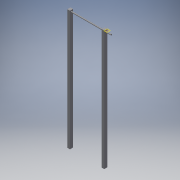
# Autodesk Inventor part: antebrazo
Saved by Autodesk Inventor 2016 (Build 200138000, 138)
## iProperties
Created: 2016-07-27
Part Number: antebrazo
Material: Generic
Document SubType Name: Modeling
Designer: Admin
Density: 1 g/cm^3
Appearance: Default
Author: Admin
Autodesk Inventor part; units mm, degrees
ref_plane "YZ Plane" through (0, 0, 0) normal (1, 0, 0) x (0, 1, 0)
ref_plane "XZ Plane" through (0, 0, 0) normal (0, 1, 0) x (-1, 0, 0)
ref_plane "XY Plane" through (0, 0, 0) normal (0, 0, 1) x (1, 0, 0)
ref_plane "Work Plane1" through (816103.6043, 395739.5889, 5886.7052) normal (0, 0, 1) x (1, 0, 0)
sketch "Sketch1" plane through (816103.6043, 395739.5889, 5886.7052) normal (0, 0, 1) x (1, 0, 0)
  line L0 (-6, 7) -> (-16, 7)
  line L1 (-16, 7) -> (-16, -5)
  line L2 (-16, -5) -> (-6, -5)
  line L3 (-6, -5) -> (-6, 7)
  line L4 (-144.5049, 7) -> (-134.5049, 7)
  line L5 (-134.5049, 7) -> (-134.5049, -5)
  line L6 (-134.5049, -5) -> (-144.5049, -5)
  line L7 (-144.5049, -5) -> (-144.5049, 7)
  point P0 (-816103.6043, -395739.5889)
  dimension "d0" = 10
  dimension "d1" = 12
  dimension "d2" = 10
  dimension "d3" = 12
  constraints: 16 end point, 4 parallel, 2 horizontal, 2 perpendicular, 1 point on line
  measures "d0" distance of L2.end L1.end
  measures "d1" distance of L1.end L0.end
  measures "d2" distance of L5.end L6.end
  measures "d3" distance of L4.end L5.end
extrude "Extrusion1" add sketch "Sketch1" against normal blind 450
sketch "Sketch2" plane through (815969.0994, 395734.5889, 5886.7052) normal (1, 0, 0) x (0, 0, -1)
  circle A0 centre (6, 6) radius 2.25
  point P0 (5886.7052, -395734.5889)
  dimension "d6" = 4.5
  constraints: 1 centre point
  measures "d6" diameter of A0
extrude "Extrusion2" add sketch "Sketch2" along normal blind 130
body "Solid1"
